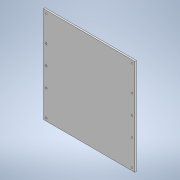
# Autodesk Inventor part: BottomPlate-4x1
Saved by Autodesk Inventor 2021 (Build 250183000, 183)
## iProperties
Created: 2020-06-16
Part Number: BottomPlate-4x1
Material: Generic
Document SubType Name: Modeling
Designer: lucas
Density: 1 g/cm^3
Appearance: Default
Author: lucas
Autodesk Inventor part; units mm, degrees
ref_plane "YZ Plane" through (0, 0, 0) normal (1, 0, 0) x (0, 1, 0)
ref_plane "XZ Plane" through (0, 0, 0) normal (0, 1, 0) x (-1, 0, 0)
ref_plane "XY Plane" through (0, 0, 0) normal (0, 0, 1) x (1, 0, 0)
sketch "Sketch1" plane through (0, 0, 0) normal (0, 0, 1) x (1, 0, 0)
  line L0 (93.3916, -12.6) -> (93.3916, 12.6)
  line L1 (53.9763, -12.6) -> (93.3916, -12.6)
  line L2 (53.9763, -15.2) -> (53.9763, -12.6)
  line L3 (38.2753, -15.2) -> (53.9763, -15.2)
  line L4 (38.2753, -15.2) -> (23.4296, -15.2)
  line L5 (23.4296, -12.6) -> (23.4296, -15.2)
  line L6 (-76.0546, -12.6) -> (23.4296, -12.6)
  line L7 (23.4296, 12.6) -> (-76.0546, 12.6)
  line L8 (23.4296, 15.2) -> (23.4296, 12.6)
  line L9 (-76.0546, 12.6) -> (-76.0546, -12.6)
  line L10 (-70.1, 10) -> (-66.9, 10)
  line L11 (-66.9, -10) -> (-70.1, -10)
  line L12 (23.4296, 15.2) -> (53.9763, 15.2)
  line L13 (53.9763, 15.2) -> (53.9763, 12.6)
  line L14 (53.9763, 12.6) -> (93.3916, 12.6)
  line L15 (-77.0546, 13.6) -> (22.4296, 13.6)
  line L16 (22.4296, 13.6) -> (22.4296, 16.2)
  line L17 (22.4296, 16.2) -> (54.9763, 16.2)
  line L18 (54.9763, 16.2) -> (54.9763, 13.6)
  line L19 (54.9763, 13.6) -> (94.3916, 13.6)
  line L20 (94.3916, 13.6) -> (94.3916, -13.6)
  line L21 (94.3916, -13.6) -> (54.9763, -13.6)
  line L22 (54.9763, -13.6) -> (54.9763, -16.2)
  line L23 (54.9763, -16.2) -> (38.2753, -16.2)
  line L24 (38.2753, -16.2) -> (22.4296, -16.2)
  line L25 (22.4296, -16.2) -> (22.4296, -13.6)
  line L26 (22.4296, -13.6) -> (-77.0546, -13.6)
  line L27 (-77.0546, -13.6) -> (-77.0546, 13.6)
  line L28 (22.4296, -16.2) -> (22.4296, -20.2) construction
  line L29 (22.4296, -20.2) -> (-87.5704, -20.2)
  line L30 (-87.5704, -20.2) -> (-87.5704, 20.2)
  line L31 (-87.5704, 20.2) -> (22.4296, 20.2)
  line L32 (104.4296, -20.2) -> (22.4296, -20.2)
  line L33 (22.4296, 20.2) -> (104.4296, 20.2)
  line L34 (104.4296, 20.2) -> (104.4296, -20.2)
  dimension "d0" = 1
  dimension "d1" = 4
  dimension "d2" = 110
  dimension "d3" = 40.4
  dimension "d5" = 82
  constraints: 70 end point, 7 perpendicular, 2 horizontal, 1 parallel, 1 point on line, 1 vertical, 12 other
  measures "d0" distance between parallel lines of L7 L15
  measures "d1" distance of L24.end L28.end
  measures "d2" distance of L28.end L29.end
  measures "d3" distance of L29.end L30.end
  measures "d5" distance of L31.end L33.end
extrude "Extrusion1" add sketch "Sketch1" against normal blind 3.5 contours L1 L2 L3 L4 L5 L6 L9 L7 L8 L12 L13 L14 L0 | L15 L16 L17 L18 L19 L20 L21 L22 L23 L24 L25 L26 L27 | L29 L30 L31 L33 L34 L32
pattern_linear "Rectangular Pattern1" count 4 spacing 40.4 along (0, -1, 0)
sketch "Sketch2" plane through (-87.5704, 20.2, 0) normal (0, 1, 0) x (1, 0, 0)
  line L0 (192, 3.5) -> (192, 0) projected
  line L1 (192, 0) -> (0, 0) projected
  line L2 (0, 0) -> (0, 3.5) projected
  line L3 (0, 3.5) -> (192, 3.5) projected
  point P0 (87.5704, 0)
extrude "Extrusion2" add sketch "Sketch2" along normal blind 20
sketch "Sketch3" plane through (-87.5704, -141.4, 0) normal (0, -1, 0) x (1, 0, 0)
  line L0 (192, 0) -> (192, -3.5) projected
  line L1 (192, -3.5) -> (0, -3.5) projected
  line L2 (0, -3.5) -> (0, 0) projected
  line L3 (0, 0) -> (192, 0) projected
  point P0 (87.5704, 0)
extrude "Extrusion3" add sketch "Sketch3" along normal blind 20
sketch "Sketch4" plane through (0, 0, -3.5) normal (0, 0, -1) x (-1, 0, 0)
  line L0 (87.5704, -161.4) -> (-104.4296, -161.4) projected
  line L1 (87.5704, -161.4) -> (81.5704, -161.4)
  line L2 (81.5704, -161.4) -> (81.5704, 40.2)
  line L3 (-104.4296, 40.2) -> (87.5704, 40.2) projected
  line L4 (81.5704, -161.4) -> (81.5704, -155.4)
  line L5 (81.5704, 40.2) -> (81.5704, 34.2)
  line L6 (77.0546, -107.6) -> (-22.4296, -107.6) projected
  line L7 (77.0546, -67.2) -> (77.0546, -94.4) projected
  line L8 (77.0546, -107.6) -> (77.0546, -94.4)
  line L9 (77.0546, -101) -> (81.5704, -101)
  line L10 (77.0546, -67.2) -> (77.0546, -53.8327)
  line L11 (77.0546, -60.5163) -> (81.5704, -60.6)
  line L12 (77.0546, -54) -> (77.0546, -26.8) projected
  line L13 (77.0546, -26.8) -> (77.0546, -13.3059)
  line L14 (77.0546, -20.0529) -> (81.5704, -20.0529)
  line L15 (-94.3916, -107.6) -> (-54.9763, -107.6) projected
  line L16 (-94.3916, -67.2) -> (-94.3916, -94.4) projected
  line L17 (-94.3916, -107.6) -> (-94.3916, -94.4)
  line L18 (-54.9763, -54) -> (-94.3916, -54) projected
  line L19 (-94.3916, -67.2) -> (-94.3916, -54)
  line L20 (-54.9763, -13.6) -> (-94.3916, -13.6) projected
  line L21 (-94.3916, -13.6) -> (-94.3916, 13.6) projected
  line L22 (-94.3916, -13.6) -> (-94.3916, 13.6)
  line L23 (-104.4296, -161.4) -> (-98.4296, -161.4)
  line L24 (-98.4296, -161.4) -> (-98.4296, 40.2)
  line L25 (-94.3916, -101) -> (-98.4296, -101)
  line L26 (-94.3916, -60.6) -> (-98.4296, -60.6)
  line L27 (-94.3916, -26.8) -> (-94.3916, -13.6)
  line L28 (-94.3916, -20.2) -> (-98.4296, -20.2)
  line L29 (-98.4296, 40.2) -> (-98.4296, 34.2)
  line L30 (-98.4296, -161.4) -> (-98.4296, -155.4)
  point P0 (0, 0)
  dimension "d15" = 6
  dimension "d16" = 6
  dimension "d17" = 6
  dimension "d18" = 6
  dimension "d19" = 6
  dimension "d20" = 6
  constraints: 42 end point, 12 point on line, 10 coincident, 8 midpoint, 6 vertical, 5 perpendicular, 2 horizontal, 1 collinear
  measures "d15" distance of L0.start L1.end
  measures "d16" distance of L1.end L4.end
  measures "d17" distance of L2.end L5.end
  measures "d18" distance of L0.end L23.end
  measures "d19" distance of L24.end L29.end
  measures "d20" distance of L23.end L30.end
hole "Hole1" at (98.4296, -155.4, -3.5) at (98.4296, -155.4, -3.5) at (98.4296, -101, -3.5) at (98.4296, -60.6, -3.5) at (98.4296, -20.2, -3.5) at (98.4296, 34.2, -3.5) at (-81.5704, 34.2, -3.5) at (-81.5704, -20.0529, -3.5) at (-81.5704, -60.6, -3.5) at (-81.5704, -101, -3.5) at (-81.5704, -155.4, -3.5) direction (0, 0, 1) diameter 3.4 end through all clearance for "Flat Head Machine Screw" size "M3" standard "Ansi Metric M Profile"
body "Solid1"
